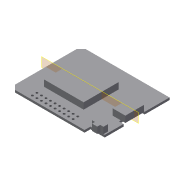
# Autodesk Inventor part: 00_ESP32_Mini
Saved by Autodesk Inventor 2019.4 (Build 234330000, 330)
## iProperties
Created: 2019-10-07
Part Number: 00_ESP32_Mini
Material: Generic
Document SubType Name: Modeling
Designer: diederichbenedict
Density: 1 g/cm^3
Appearance: Green Polished
Author: diederichbenedict
Autodesk Inventor part; units mm, degrees
ref_plane "YZ Plane" through (0, 0, 0) normal (1, 0, 0) x (0, 1, 0)
ref_plane "XZ Plane" through (0, 0, 0) normal (0, 1, 0) x (-1, 0, 0)
ref_plane "XY Plane" through (0, 0, 0) normal (0, 0, 1) x (1, 0, 0)
sketch "Sketch1" plane through (0, 0, 0) normal (0, 1, 0) x (-1, 0, 0)
  line L0 (0, -2) -> (0, -29.2)
  line L1 (-2, -31.2) -> (-39, -31.2)
  line L2 (-39, -31.2) -> (-39, -20.2)
  line L3 (-39, -20.2) -> (-37, -20.2)
  line L4 (-37, -20.2) -> (-37, -10.9)
  line L5 (-37, -10.9) -> (-39, -10.9)
  line L6 (-39, -10.9) -> (-39, -2.6)
  line L7 (-39, -2.6) -> (-32.7, -2.6)
  line L8 (-32.7, -2.6) -> (-32.7, 0)
  line L9 (-32.7, 0) -> (-2, 0)
  line L10 (0, -2) -> (-2, 0)
  line L11 (0, -29.2) -> (-2, -31.2)
  point P0 (0, 0)
  point P1 (0, -31.2)
  dimension "d0" = 31.2
  dimension "d1" = 39
  dimension "d2" = 11
  dimension "d3" = 2
  dimension "d4" = 9.3
  dimension "d5" = 8.3
  dimension "d6" = 6.3
  dimension "d7" = 2
  dimension "d8" = 2
  dimension "d9" = 2
  dimension "d10" = 2
  constraints: 24 end point, 8 perpendicular, 4 point on line, 1 horizontal, 1 vertical
  measures "d0" distance of point (0, 0) point (0, -31.2)
  measures "d1" distance of point (0, -31.2) L1.end
  measures "d2" distance of L1.end L2.end
  measures "d3" distance of L2.end L3.end
  measures "d4" distance of L3.end L4.end
  measures "d5" distance of L5.end L6.end
  measures "d6" distance of L6.end L7.end
  measures "d7" distance of L0.start point (0, 0)
  measures "d8" distance of L9.end point (0, 0)
  measures "d9" distance of L0.end point (0, -31.2)
  measures "d10" distance of L1.start point (0, -31.2)
extrude "Extrusion1" add sketch "Sketch1" along normal blind 1
sketch "Sketch2" plane through (0, 1, 0) normal (0, 1, 0) x (1, 0, 0)
  line L0 (39, 31.2) -> (2, 31.2) projected
  line L1 (2, 31.2) -> (0, 29.2) projected
  line L2 (0, 29.2) -> (0, 2) projected
  line L3 (0, 2) -> (2, 0) projected
  line L4 (2, 0) -> (32.7, 0) projected
  line L5 (32.7, 0) -> (32.7, 2.6) projected
  line L6 (32.7, 2.6) -> (39, 2.6) projected
  line L7 (39, 2.6) -> (39, 10.9) projected
  line L8 (39, 10.9) -> (37, 10.9) projected
  line L9 (37, 10.9) -> (37, 20.2) projected
  line L10 (37, 20.2) -> (39, 20.2) projected
  line L11 (39, 20.2) -> (39, 31.2) projected
  line L12 (7.2, 7.6) -> (24.7, 7.6)
  line L13 (24.7, 7.6) -> (24.7, 23.1)
  line L14 (24.7, 23.1) -> (7.2, 23.1)
  line L15 (7.2, 23.1) -> (7.2, 7.6)
  line L16 (39, 11.7) -> (33.4, 11.7)
  line L17 (33.4, 11.7) -> (33.4, 19.9)
  line L18 (33.4, 19.9) -> (39, 19.9)
  line L19 (39, 19.9) -> (39, 11.7)
  line L20 (32.7, 2.6) -> (39, 2.6) projected
  line L21 (33.4, 4.6553) -> (38.4269, 4.6553)
  line L22 (38.4269, 4.6553) -> (38.4269, 2.6)
  line L23 (38.4269, 2.6) -> (33.4, 2.6)
  line L24 (33.4, 2.6) -> (33.4, 4.6553)
  line L25 (34.7176, 2.6) -> (37, 2.6)
  line L26 (37, 2.6) -> (37, 1.3)
  line L27 (37, 1.3) -> (34.7176, 1.3)
  line L28 (34.7176, 1.3) -> (34.7176, 2.6)
  point P0 (0, 0)
  dimension "d13" = 17.5
  dimension "d14" = 15.5
  dimension "d15" = 7.6
  dimension "d16" = 7.2
  dimension "d17" = 5.6
  dimension "d18" = 8.2
  dimension "d19" = 11.7
  constraints: 32 end point, 8 parallel, 4 horizontal, 4 perpendicular, 2 point on line
  measures "d13" distance of L14.end L13.end
  measures "d14" distance of L13.end L12.end
  measures "d15" distance between parallel lines of L12 L4
  measures "d16" distance between parallel lines of L15 L2
  measures "d17" distance of L17.end L18.end
  measures "d18" distance of L16.end L17.end
  measures "d19" distance between parallel lines of L16 L4
extrude "Extrusion2" add sketch "Sketch2" along normal blind 2.8 contours L18 L19 L16 L9 | L9 L16 L17 L18 | L24 L21 L22 L6 | L6 L26 L27 L28 | L15 L14 L13 L12
sketch "Sketch3" plane through (0, 1, 0) normal (0, 1, 0) x (1, 0, 0)
  line L0 (2, 0) -> (32.7, 0) projected
  line L1 (0, 29.2) -> (0, 2) projected
  point P0 (0, 0)
  point P1 (8, 1.7)
  dimension "d22" = 1.7
  dimension "d23" = 8
  measures "d22" distance from line of point (8, 1.7) L0
  measures "d23" distance from line of point (8, 1.7) L1
hole "Hole1" at (8, 1, -1.7) direction (0, -1, 0) diameter 1 depth 16 tip angle 118
pattern_linear "Rectangular Pattern1" count 10 spacing 2 along (1, 0, 0) of "Hole1"
pattern_linear "Rectangular Pattern2" count 2 spacing 2 along (0, 0, -1) of "Hole1", "Rectangular Pattern1"
ref_plane "Work Plane1" through (2, 0, -15.6) normal (0, 0, 1) x (1, 0, 0)
mirror "Mirror1" [suppressed]
sketch "Sketch4" plane through (2, 0, 0) normal (0, 0, 1) x (1, 0, 0)
  line L0 (5.5, 0) -> (5.5, 1) projected
  line L1 (6.5, 0) -> (6.5, 1) projected
  circle A0 centre (6, 2.25) radius 0.5
  line L2 (0, 1) -> (30.7, 1) projected
  line L3 (5.25, 3) -> (6.75, 3)
  line L4 (6.75, 3) -> (6.75, 1.5)
  line L5 (6.75, 1.5) -> (5.25, 1.5)
  line L6 (5.25, 1.5) -> (5.25, 3)
  line L7 (5.25, 3) -> (6.75, 1.5) construction
  line L8 (6.75, 3) -> (5.25, 1.5) construction
  point P0 (-2, 0)
  dimension "d37" = 1.25
  dimension "d42" = 1.5
  dimension "d43" = 1.5
  constraints: 12 end point, 2 midpoint, 2 parallel, 2 tangent, 1 centre point, 1 horizontal, 1 perpendicular
  measures "d37" distance from line of A0.centre L2
  measures "d42" distance of L4.end L5.end
  measures "d43" distance of L3.end L4.end
extrude "Extrusion3" [suppressed]
pattern_linear "Rectangular Pattern3" [suppressed]
mirror "Mirror2" [suppressed]
equation "\"d8\" = d7"
equation "\"d9\" = d7"
equation "\"d10\" = d9"
body "Solid1"
